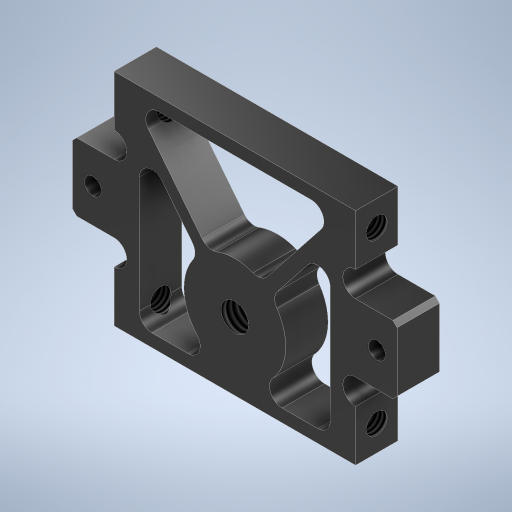
# Autodesk Inventor part: LegBaseFrontFulcrumFrame
Saved by Autodesk Inventor 2024.2 (Build 282272000, 272)
## iProperties
Created: 2024-01-07
Part Number: LegBaseFrontFulcrumFrame
Material: Aluminum 7075
Document SubType Name: Modeling
Designer: Masato Kubotera
Density: 2.81 g/cm^3
Appearance: Glossy - Black
Vendor: meviy
Mass: 7.31604 g
Surface Area: 27.2207 cm^2
Volume: 2.60357 cm^3
Author: Masato Kubotera
Autodesk Inventor part; units mm, degrees
ref_plane "YZ Plane" through (0, 0, 0) normal (1, 0, 0) x (0, 1, 0)
ref_plane "XZ Plane" through (0, 0, 0) normal (0, 1, 0) x (-1, 0, 0)
ref_plane "XY Plane" through (0, 0, 0) normal (0, 0, 1) x (1, 0, 0)
sketch "Sketch1" plane through (0, 0, 0) normal (1, 0, 0) x (0, 1, 0)
  line L0 (0, 12.5) -> (0, -8) construction
  line L1 (-14.25, 18) -> (14.25, 18)
  line L2 (14.25, 18) -> (14.25, 9)
  line L3 (14.25, 9) -> (19.15, 9)
  line L4 (19.15, 9) -> (19.15, 1)
  line L5 (19.15, 1) -> (14.25, 1)
  line L6 (14.25, 1) -> (14.25, -8)
  line L7 (14.25, -8) -> (-14.25, -8)
  arc A0 (14.25, 12) -> (14.25, 9) centre (14.25, 10.5) ccw
  line L8 (19.15, 5) -> (-19.15, 5) construction
  arc A1 (14.25, 1) -> (14.25, -2) centre (14.25, -0.5) ccw
  line L9 (-14.25, 18) -> (-14.25, 9)
  line L10 (-14.25, 9) -> (-19.15, 9)
  line L11 (-19.15, 9) -> (-19.15, 1)
  line L12 (-19.15, 1) -> (-14.25, 1)
  line L13 (-14.25, 1) -> (-14.25, -8)
  arc A2 (-14.25, 9) -> (-14.25, 12) centre (-14.25, 10.5) ccw
  arc A3 (-14.25, -2) -> (-14.25, 1) centre (-14.25, -0.5) ccw
  line L14 (14.25, -5) -> (8.25, -5) construction
  line L15 (-14.25, -5) -> (-8.25, -5) construction
  circle A4 centre (0, 0) radius 6 construction
  line L16 (14.25, 18) -> (0, 0) construction
  line L17 (0, 0) -> (14.25, -8) construction
  line L18 (-9.0053, 16.5) -> (9.0053, 16.5)
  line L19 (10.1813, 14.0689) -> (3.8528, 6.075)
  line L20 (-10.1813, 14.0689) -> (-3.8528, 6.075)
  line L21 (8.5739, 9.6219) -> (5.0289, 5.144)
  line L22 (11.25, -5) -> (11.25, 8.6909)
  arc A5 (2.1414, 5.6049) -> (-2.1414, 5.6049) centre (0, 0) ccw
  arc A6 (4.4721, -4) -> (4.964, 3.3703) centre (0, 0) ccw
  arc A7 (-9.0053, 16.5) -> (-10.1813, 14.0689) centre (-9.0053, 15) ccw
  arc A8 (-3.8528, 6.075) -> (-2.1414, 5.6049) centre (-2.6767, 7.0061) ccw
  arc A9 (2.1414, 5.6049) -> (3.8528, 6.075) centre (2.6767, 7.0061) ccw
  arc A10 (10.1813, 14.0689) -> (9.0053, 16.5) centre (9.0053, 15) ccw
  arc A11 (11.25, 8.6909) -> (8.5739, 9.6219) centre (9.75, 8.6909) ccw
  arc A12 (9.75, -6.5) -> (11.25, -5) centre (9.75, -5) ccw
  arc A13 (5.0289, 5.144) -> (4.964, 3.3703) centre (6.2049, 4.2129) ccw
  line L23 (-8.5739, 9.6219) -> (-5.0289, 5.144)
  line L24 (-11.25, -5) -> (-11.25, 8.6909)
  arc A14 (-4.964, 3.3703) -> (-4.4721, -4) centre (0, 0) ccw
  arc A15 (-8.5739, 9.6219) -> (-11.25, 8.6909) centre (-9.75, 8.6909) ccw
  arc A16 (-4.964, 3.3703) -> (-5.0289, 5.144) centre (-6.2049, 4.2129) ccw
  line L25 (16.75, 9) -> (16.75, 1) construction
  line L26 (9.75, -6.5) -> (5.5902, -6.5)
  arc A17 (4.4721, -4) -> (5.5902, -6.5) centre (5.5902, -5) ccw
  arc A18 (-11.25, -5) -> (-9.75, -6.5) centre (-9.75, -5) ccw
  line L27 (-9.75, -6.5) -> (-5.5902, -6.5)
  arc A19 (-5.5902, -6.5) -> (-4.4721, -4) centre (-5.5902, -5) ccw
  line L28 (14.25, 15) -> (8.25, 15) construction
  point P0 (-14.25, -2)
  point P1 (14.25, -2)
  point P2 (-16.75, 5)
  point P3 (12.1059, 16.5)
  point P4 (3.107, 5.1329)
  point P5 (-12.1059, 16.5)
  point P6 (-3.107, 5.1329)
  point P7 (4.283, 4.2019)
  point P8 (16.75, 5)
  dimension "d6" = 9
  dimension "d7" = 1.5
  dimension "d8" = 8
  dimension "d9" = 4.9
  dimension "d10" = 28.5
  dimension "d18" = 9
  dimension "d19" = 6
  dimension "d20" = 6
  dimension "d60" = 12
  dimension "d62" = 1.5
  dimension "d66" = 1.5
  dimension "d74" = 1.5
  dimension "d77" = 18
  dimension "d78" = 2.5
  dimension "d79" = 3
  constraints: 58 end point, 44 point on circle, 31 symmetric about line, 20 centre point, 16 tangent, 14 point on line, 7 equal radius, 7 horizontal, 4 coincident, 4 midpoint, 4 vertical, 2 parallel, 1 collinear, 10 other
  measures "d6" distance between parallel lines of L3 L1
  measures "d7" radius of A0
  measures "d8" distance of L3.end L4.end
  measures "d9" distance of L2.end L3.end
  measures "d10" distance of L1.start L1.end
  measures "d18" distance between parallel lines of L7 L5
  measures "d19" distance of L14.start L14.end
  measures "d20" distance between parallel lines of L14 L5
  measures "d60" diameter of A4
  measures "d62" distance between parallel lines of L21 L19
  measures "d66" radius of A7
  measures "d74" distance between parallel lines of L7 L26
  measures "d77" distance from line of point (0, 0) L1
  measures "d78" distance between parallel lines of L2 L25
  measures "d79" distance between parallel lines of L6 L22
extrude "Extrusion1" add sketch "Sketch1" against normal blind 5 contours L1 L2 A0 L3 L4 L5 A1 L6 L7 L13 A3 L12 L11 L10 A2 L9
hole "M4" at (0, 0, 0) direction (-1, 0, 0) diameter 3.242 end through all thread size "M4x0.7" class "6H" standard "ANSI Metric M Profile"
sketch "Sketch2" plane through (0, 14.25, -2) normal (0, 1, 0) x (1, 0, 0)
  line L0 (-5, -11) -> (-5, -20) projected
  line L1 (0, 3) -> (-5, 3) construction
  line L2 (-5, -3) -> (-5, 6) projected
  line L3 (-5, -17) -> (0, -17) construction
  line L4 (0, -14) -> (0, -20) projected
  point P0 (0, -2)
  point P1 (-5, -14)
  point P2 (-5, 0)
  point P3 (-2.5, 3)
  point P4 (-2.5, -17)
  point P5 (0, -17)
  point P6 (0, -17)
  constraints: 4 end point, 3 midpoint, 2 horizontal, 2 point on line
hole "Side-M3" at (-2.5, 14.25, -5) at (-2.5, 14.25, 15) direction (0, -1, 0) diameter 2.459 depth 6 thread size "M3x0.5" class "6H" standard "ANSI Metric M Profile"
hole "Phi2-H7" at (0, -16.75, 5) at (0, 16.75, 5) direction (-1, 0, 0) diameter 2 end through all
mirror "Mirror1" about plane through (0, 0, 0) normal (0, 1, 0) of "Side-M3"
chamfer "0.5" distance 0.5 angle 45 4 edges at (-2.5, 19.15, 9) (-2.5, 19.15, 1) (-2.5, -19.15, 9) (-2.5, -19.15, 1)
equation "\"d35\" = d19"
body "Solid1"
